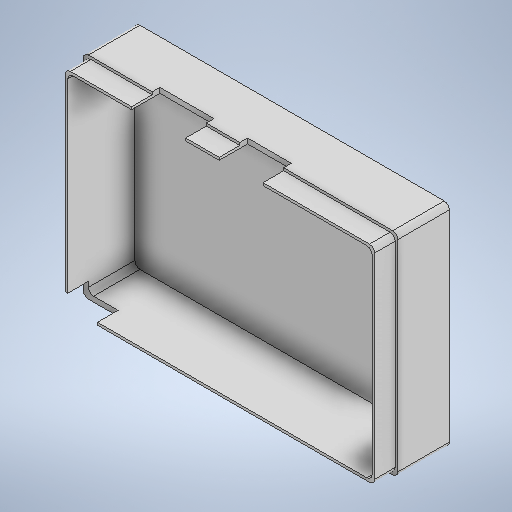
# Autodesk Inventor part: caixa_KiiRA
Saved by Autodesk Inventor 2026.3 (Build 303398000, 398)
## iProperties
Created: 2026-05-20
Part Number: caixa_KiiRA
Material: Genérico
Document SubType Name: Modeling
Designer: franciscowilke
Density: 1 g/cm^3
Appearance: Padrão
Author: franciscowilke
Autodesk Inventor part; units mm, degrees
ref_plane "YZ Plane" through (0, 0, 0) normal (1, 0, 0) x (0, 1, 0)
ref_plane "XZ Plane" through (0, 0, 0) normal (0, 1, 0) x (-1, 0, 0)
ref_plane "XY Plane" through (0, 0, 0) normal (0, 0, 1) x (1, 0, 0)
sketch "Esboço1" plane through (0, 0, 0) normal (0, 0, 1) x (1, 0, 0)
  line L0 (-59, 39) -> (59, 39)
  line L1 (59, 39) -> (59, -39)
  line L2 (59, -39) -> (-59, -39)
  line L3 (-59, -39) -> (-59, 39)
  line L4 (-59, 39) -> (59, -39) construction
  line L5 (59, 39) -> (-59, -39) construction
  line L6 (60, 40) -> (-60, 40)
  line L7 (-60, 40) -> (-60, -40)
  line L8 (-60, -40) -> (60, -40)
  line L9 (60, -40) -> (60, 40)
  line L10 (-61, 41) -> (61, 41)
  line L11 (61, 41) -> (61, -41)
  line L12 (61, -41) -> (-61, -41)
  line L13 (-61, -41) -> (-61, 41)
  point P0 (0, 0)
  dimension "d14" = 118
  dimension "d15" = 78
  dimension "d16" = 1
  dimension "d17" = 1
  constraints: 28 end point, 6 parallel, 3 perpendicular, 2 midpoint, 1 horizontal, 6 other
  measures "d14" distance of L0.start L0.end
  measures "d15" distance of L0.end L1.end
  measures "d16" distance between parallel lines of L8 L2
  measures "d17" distance between parallel lines of L12 L8
extrude "Extrusão8" add sketch "Esboço1" against normal blind 20 contours L0 L1 L2 L3 | L9 L8 L7 L6 | L10 L11 L12 L13
extrude "Extrusão9" cut sketch "Esboço1" against normal blind 18 contours L0 L1 L2 L3
extrude "Extrusão10" add sketch "Esboço1" along normal blind 8 contours L9 L8 L7 L6
fillet "Arredondamento4" radius 2 12 edges at (61, 41, -10) (60, 40, 4) (61, -41, -10) (60, -40, 4) (-61, 41, -10) (-60, 40, 4) (-60, -40, 4) (-61, -41, -10) (59, 39, -5) (-59, 39, -5) (59, -39, -5) (-59, -39, -5)
sketch "Esboço4" plane through (-59, 41, 0) normal (0, 1, 0) x (1, 0, 0)
  line L0 (120, 0) -> (120, 20) construction
  line L1 (2, -8) -> (116, -8) construction
  line L2 (75.727, -8) -> (58.727, -8)
  line L3 (58.727, -8) -> (58.727, 3)
  line L4 (58.727, 3) -> (75.727, 3)
  line L5 (75.727, 3) -> (75.727, -8)
  line L6 (45.727, -8) -> (24.727, -8)
  line L7 (24.727, -8) -> (24.727, 3)
  line L8 (24.727, 3) -> (45.727, 3)
  line L9 (45.727, 3) -> (45.727, -8)
  point P0 (59, 0)
  dimension "d46" = 11
  dimension "d48" = 21
  dimension "d49" = 17
  constraints: 16 end point, 4 parallel, 2 horizontal, 2 perpendicular, 1 point on line
  measures "d46" distance of L8.end L6.start
  measures "d48" distance of L7.end L8.end
  measures "d49" distance of L3.end L4.end
extrude "Extrusão11" cut sketch "Esboço4" against normal blind 4
sketch "Esboço9" plane through (-59, -41, 0) normal (0, -1, 0) x (1, 0, 0)
  line L0 (-2, 0) -> (-2, -20) construction
  line L1 (-2, 0) -> (11.5, 0)
  line L2 (11.5, 0) -> (11.5, 8)
  line L3 (11.5, 8) -> (-2, 8)
  line L4 (-2, 8) -> (-2, 0)
  point P0 (59, 0)
  dimension "d62" = 13.5
  dimension "d63" = 8
  constraints: 8 end point, 2 parallel, 1 horizontal, 1 perpendicular, 1 point on line
  measures "d62" distance of L3.end L2.end
  measures "d63" distance of L2.end L1.end
extrude "Extrusão14" cut sketch "Esboço9" against normal blind 6
